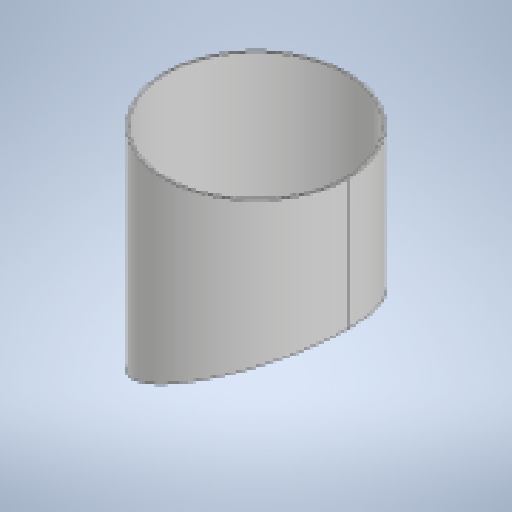
# Autodesk Inventor part: GBK-RK-0031 tube segmeng 1
Saved by Autodesk Inventor 2026.2 (Build 302298000, 298)
## iProperties
Created: 2026-09-14
Part Number: GBK-RK-0031 tube segmeng 1
Material: Generic
Document SubType Name: Sheet Metal
Designer: admin
Density: 1 g/cm^3
Flat Pattern Width: 40 cm
Flat Pattern Length: 101.018 cm
Flat Pattern Area: 4040.72 cm^2
Sheet Metal Rule: Default_mm
Sheet Metal Width: 400,000 mm
Sheet Metal Length: 1010,181 mm
Sheet Metal Area: 404072,471 mm^2
Appearance: Default
Author: admin
Autodesk Inventor part; units mm, degrees
ref_plane "YZ Plane" through (0, 0, 0) normal (1, 0, 0) x (0, 1, 0)
ref_plane "XZ Plane" through (0, 0, 0) normal (0, 1, 0) x (-1, 0, 0)
ref_plane "XY Plane" through (0, 0, 0) normal (0, 0, 1) x (1, 0, 0)
sketch "Sketch1" plane through (0, 0, 0) normal (0, 0, 1) x (1, 0, 0)
  line L0 (0, 0) -> (0, 204.8418)
  line L1 (159.5, 0) -> (162.5, 0)
  line L2 (162.5, 0) -> (162.5, 400)
  line L3 (162.5, 400) -> (159.5, 400)
  line L4 (159.5, 400) -> (159.5, 0)
  dimension "d0" = 3
  dimension "d1" = 400
  dimension "d2" = 325
  constraints: 10 end point, 2 parallel, 1 horizontal, 1 perpendicular, 1 point on line, 1 vertical
  measures "d0" distance of L3.end L2.end
  measures "d1" distance of L2.end L1.end
  measures "d2" diameter of L2 L0
revolve "Revolution1" add sketch "Sketch1" angle 359.9 about axis through (0, 0, 0) along (0, 1, 0)
sketch "Sketch2" plane through (0, 0, 0) normal (0, 0, 1) x (1, 0, 0)
  line L0 (162.5, 400) -> (-162.5, 400) construction
  line L1 (162.5, 0) -> (162.5, 400) projected
  line L2 (-162.5, 0) -> (-162.5, 400) projected
  line L3 (162.5, 0) -> (-162.5, 0) projected
  line L4 (-162.5, 0) -> (162.5, 70.6832)
  point P0 (0, 0)
  point P1 (162.4998, 400)
  point P2 (162.4998, 0)
  dimension "d6" = 12.27
  constraints: 2 end point, 1 point on line
  measures "d6" angle of L3 L4
extrude "Extrusion1" cut sketch "Sketch2" along normal through all both and the other way through all
equation "\"BendRadius\" = Thickness"
equation "\"BendReliefWidth\" = Thickness"
equation "\"BendReliefDepth\" = 0.5 * Thickness"
equation "\"CornerReliefSize\" = 4 * Thickness"
equation "\"MinimumRemnant\" = 2 * Thickness"
equation "\"TransitionRadius\" = BendRadius"
equation "\"JacobiRadiusSize\" = BendRadius"
equation "\"GapSize\" = Thickness"
equation "\"Thickness\" = 3"
body "Solid1"
